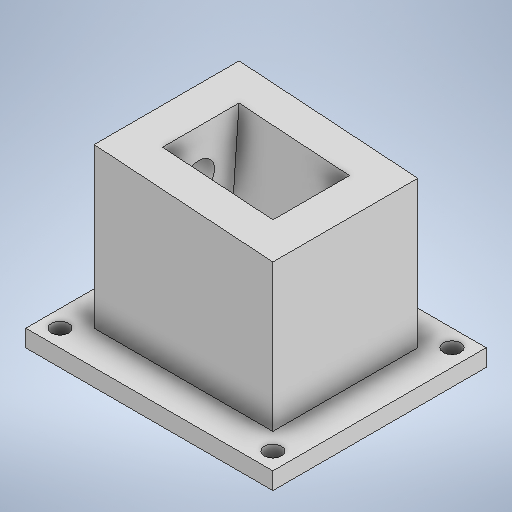
# Autodesk Inventor part: sort support V3
Saved by Autodesk Inventor 2025.3 (Build 293356000, 356)
## iProperties
Created: 2026-05-01
Part Number: sort support V3
Material: Generic
Document SubType Name: Modeling
Designer: kamal
Density: 1 g/cm^3
Appearance: Default
Author: kamal
## iProperties of the stored document sort support V3_3DPrint.ipt
Created: 2026-05-01
Part Number: sort support V3_3DPrint
Material: Generic
Document SubType Name: Modeling
Designer: kamal
Density: 1 g/cm^3
Appearance: Default
Author: kamal
Autodesk Inventor part; units mm, degrees
ref_plane "YZ Plane" through (0, 0, 0) normal (1, 0, 0) x (0, 1, 0)
ref_plane "XZ Plane" through (0, 0, 0) normal (0, 1, 0) x (-1, 0, 0)
ref_plane "XY Plane" through (0, 0, 0) normal (0, 0, 1) x (1, 0, 0)
sketch "Sketch1" plane through (0, 0, 0) normal (0, 0, 1) x (1, 0, 0)
  line L0 (0, 0) -> (0, 46.52)
  line L1 (0, 46.52) -> (52.2762, 42.9195)
  line L2 (52.2762, 42.9195) -> (52.2762, 0)
  line L3 (52.2762, 0) -> (0, 0)
  dimension "d0" = 46.52
  dimension "d1" = 52.4
  dimension "d2" = 86.06
  constraints: 8 end point, 2 vertical, 1 perpendicular
  measures "d0" distance of L0.start L0.end
  measures "d1" distance of L0.end L1.end
  measures "d2" angle of L0 L1
extrude "Extrusion1" add sketch "Sketch1" along normal blind 42.4
sketch "Sketch2" plane through (0, 0, 0) normal (0, -1, 0) x (1, 0, 0)
  line L0 (0, 0) -> (52.2762, 0) projected
  line L1 (52.2762, 0) -> (52.2762, 42.4) projected
  line L2 (0, 42.4) -> (52.2762, 42.4) projected
  line L3 (0, 0) -> (0, 42.4) projected
  line L4 (47.2762, 37.4) -> (47.2762, 5)
  line L5 (47.2762, 5) -> (5, 5)
  line L6 (5, 5) -> (5, 37.4)
  line L7 (5, 37.4) -> (47.2762, 37.4)
  line L8 (62.2762, 52.4) -> (62.2762, -10)
  line L9 (62.2762, -10) -> (-10, -10)
  line L10 (-10, -10) -> (-10, 52.4)
  line L11 (-10, 52.4) -> (62.2762, 52.4)
  line L12 (57.2762, 47.4) -> (57.2762, -5) construction
  line L13 (57.2762, -5) -> (-5, -5) construction
  line L14 (-5, -5) -> (-5, 47.4) construction
  line L15 (-5, 47.4) -> (57.2762, 47.4) construction
  circle A0 centre (57.2762, 47.4) radius 2.5
  circle A1 centre (-5, 47.4) radius 2.5
  circle A2 centre (-5, -5) radius 2.5
  circle A3 centre (57.2762, -5) radius 2.5
  dimension "d5" = 5
  dimension "d6" = 10
  dimension "d7" = 5
  dimension "d8" = 5
  dimension "d9" = 5
  dimension "d10" = 5
  dimension "d11" = 5
  constraints: 24 end point, 4 centre point, 4 coincident, 9 other
  measures "d5" distance between parallel lines of L1 L4
  measures "d6" distance between parallel lines of L1 L8
  measures "d7" distance between parallel lines of L1 L12
  measures "d8" diameter of A0
  measures "d9" diameter of A1
  measures "d10" diameter of A2
  measures "d11" diameter of A3
extrude "Extrusion2" add sketch "Sketch2" along normal blind 5 contours L3 L2 L1 L0 | L8 L9 L10 L11
sketch "Sketch3" plane through (0, 46.52, 42.4) normal (0.0687, 0.9976, 0) x (0.9976, -0.0687, 0)
  line L0 (42.4, 32.4) -> (10, 32.4)
  line L1 (10, 32.4) -> (10, 10)
  line L2 (10, 10) -> (42.4, 10)
  line L3 (42.4, 10) -> (42.4, 32.4)
  line L4 (42.4, 32.4) -> (10, 10) construction
  line L5 (10, 32.4) -> (42.4, 10) construction
  line L6 (52.4, 0) -> (0, 0) projected
  line L7 (0, 42.4) -> (0, 0) projected
  point P0 (3.1965, 42.4)
  point P1 (26.2, 21.2)
  dimension "d14" = 32.4
  dimension "d15" = 22.4
  dimension "d16" = 21.2
  dimension "d17" = 26.2
  constraints: 12 end point, 2 midpoint, 2 parallel, 1 horizontal, 1 perpendicular
  measures "d14" distance of L2.end L1.end
  measures "d15" distance of L0.end L1.end
  measures "d16" distance from line of L6 point (26.2, 21.2)
  measures "d17" distance from line of L7 point (26.2, 21.2)
extrude "Extrusion3" cut sketch "Sketch3" against normal through all
sketch "Sketch4" plane through (0, 46.52, 0) normal (-1, 0, 0) x (0, 0, 1)
  circle A0 centre (21.2, -15) radius 5
  line L0 (0, 0) -> (42.4, 0) projected
  line L1 (0, 0) -> (0, -46.52) projected
  dimension "d20" = 10
  dimension "d21" = 15
  dimension "d22" = 21.2
  constraints: 1 centre point
  measures "d20" diameter of A0
  measures "d21" distance from line of L0 A0.centre
  measures "d22" distance from line of L1 A0.centre
extrude "Extrusion4" cut sketch "Sketch4" against normal blind 10
body "Solid1"
